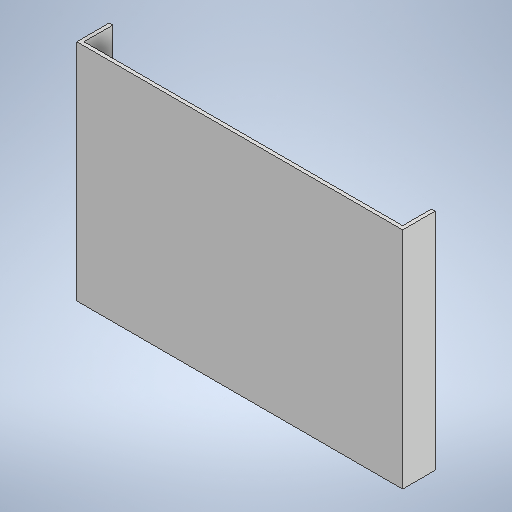
# Autodesk Inventor part: TesteProteção
Saved by Autodesk Inventor 2025.3 (Build 293356030, 356C)
## iProperties
Created: 2025-11-04
Part Number: TesteProteção
Material: Genérico
Document SubType Name: Modeling
Designer: Rubens
Density: 1 g/cm^3
Appearance: Padrão
Author: Rubens
Autodesk Inventor part; units mm, degrees
ref_plane "YZ Plane" through (0, 0, 0) normal (1, 0, 0) x (0, 1, 0)
ref_plane "XZ Plane" through (0, 0, 0) normal (0, 1, 0) x (-1, 0, 0)
ref_plane "XY Plane" through (0, 0, 0) normal (0, 0, 1) x (1, 0, 0)
sketch "Esboço1" plane through (0, 0, 0) normal (0, 0, 1) x (1, 0, 0)
  line L0 (0, 0) -> (440, 0)
  line L1 (440, 0) -> (440, 310)
  line L2 (440, 310) -> (0, 310)
  line L3 (0, 310) -> (0, 0)
  line L4 (440, 310) -> (445, 310)
  line L5 (445, 310) -> (445, 0)
  line L6 (445, 0) -> (440, 0)
  line L7 (0, 310) -> (-5, 310)
  line L8 (-5, 310) -> (-5, 0)
  line L9 (-5, 0) -> (0, 0)
  dimension "d0" = 440
  dimension "d1" = 310
  dimension "d2" = 5
  dimension "d3" = 5
  constraints: 20 end point, 5 perpendicular, 3 horizontal, 2 parallel
  measures "d0" distance of L2.end L1.end
  measures "d1" distance of L1.end L0.end
  measures "d2" distance of L1.end L4.end
  measures "d3" distance of L2.end L7.end
extrude "Extrusão1" add sketch "Esboço1" along normal blind 5
extrude "Extrusão2" add sketch "Esboço1" against normal blind 40 contours L9 L8 L7 L3 | L1 L4 L5 L6
